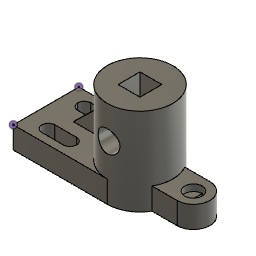
drawing_7 v1 (Autodesk Fusion 360 design; units mm, degrees)
Autodesk Fusion 360 part; units mm, degrees
sketch "Sketch10" plane through (0, 0, 0) normal (0, 1, 0) x (1, 0, 0)
  line L0 (15, -15) -> (101, -15)
  line L1 (101, -15) -> (101, -75)
  line L2 (101, -75) -> (15, -75)
  line L3 (15, -75) -> (15, -15)
  line L4 (15, -15) -> (150, -15)
  line L5 (135, -30) -> (90, -30)
  line L6 (90, -30) -> (90, -60)
  line L7 (90, -60) -> (135, -60)
  line L8 (150, -45) -> (150, -45)
  line L9 (135, -30) -> (150, -30)
  line L10 (135, -60) -> (150, -60)
  line L11 (165, -45) -> (165, -45)
  arc A0 (165, -45) -> (150, -30) centre (150, -45) ccw
  arc A1 (150, -60) -> (165, -45) centre (150, -45) ccw
  point P0 (150, -30)
  point P1 (150, -60)
  point P2 (165, -30)
  dimension "d50" = 86
  dimension "d51" = 60
  dimension "d59" = 135
  dimension "d60" = 60
  dimension "d61" = 30
  dimension "d64" = 30
  dimension "d65" = 15
  dimension "d66" = 15
  constraint horizontal L0
  constraint vertical L1
  constraint horizontal L2
  constraint vertical L3
  constraint perpendicular L3 L4
  constraint horizontal L5
  constraint vertical L6
  constraint horizontal L7
  constraint coincident P1 L7
  constraint coincident P0 L5
  constraint coincident P0 L8
  constraint horizontal L9
  constraint perpendicular L1 L10
  constraint coincident P2 L9
  constraint tangent L9 A0
  constraint tangent L10 A1
  measures "d50" distance of L0.start L0.end
  measures "d51" distance of L0.start L2.end
  measures "d59" distance of L0.start L4.end
  measures "d60" distance of P0 L5.end
  measures "d61" distance of P0 P1
  measures "d64" distance of L5.start P2
  measures "d65" radius of A0
  measures "d66" radius of A1
extrude "Extrude9" add sketch "Sketch10" along normal blind 20 contours L1 L5 L7 L9 L10 A0 A1 makes body 1
extrude "Extrude7" add sketch "Sketch10" along normal blind 20 separate body contours L0 L1 L2 L3 L4 L5 L6 L7 | L1 L5 L6 L7 makes body 2
sketch "Sketch11" plane through (0, 20, 0) normal (0, 1, 0) x (-1, 0, 0)
  line L0 (-15, 75) -> (-101, 75)
  line L1 (-101, 15) -> (-15, 15)
  line L2 (-15, 15) -> (-15, 75)
  circle A0 centre (-101, 45) radius 30
  line L3 (-101, 75) -> (-101, 15)
  dimension "d56" = 60
  measures "d56" diameter of A0
extrude "Extrude8" add sketch "Sketch11" along normal blind 60 contours A0 L3 | A0 L3 bodies 2
extrude "Extrude10" add 1 faces at (110.7493, 20, 47.2252) along direction (0, -1, 0) blind 20 on bodies 2 bodies 2 1
hole "Hole2" at (150, 20, 45) direction (0, -1, 0) diameter 16 depth 6 tip angle 180 bodies 2
sketch "Sketch12" plane through (0, 14, 0) normal (0, 1, 0) x (-1, 0, 0)
  circle A0 centre (-150, 45) radius 8
  line L0 (-150, 45) -> (-150, 37)
  line L1 (-150, 53) -> (-150, 44.4866)
  constraint coincident A0.centre L0.start
  constraint coincident A0 L0.end
  constraint vertical L0
  constraint coincident A0 L1.start
  constraint coincident L0 L1.end
  constraint parallel L0 L1
extrude "Extrude11" cut sketch "Sketch12" against normal blind 40 contours A0 L0 L1 picked at (-153.316, 49.1581) bodies 2
sketch "Sketch13" plane through (0, 80, 0) normal (0, 1, 0) x (-1, 0, 0)
  circle A0 centre (-101, 45) radius 30
  line L0 (-101, 45) -> (-91, 45)
  line L1 (-91, 45) -> (-91, 35)
  line L2 (-91, 35) -> (-101, 35)
  line L3 (-101, 35) -> (-101, 45)
  line L4 (-91, 35) -> (-111, 35)
  line L5 (-111, 35) -> (-111, 55)
  line L6 (-111, 55) -> (-91, 55)
  line L7 (-91, 55) -> (-91, 35)
  dimension "d76" = 10
  dimension "d77" = 10
  dimension "d78" = 20
  dimension "d79" = 20
  constraint horizontal L0
  constraint vertical L1
  constraint horizontal L2
  constraint vertical L3
  constraint coincident A0.centre L0.start
  constraint horizontal L4
  constraint vertical L5
  constraint horizontal L6
  constraint vertical L7
  measures "d76" distance of A0.centre L0.end
  measures "d77" distance of A0.centre L2.end
  measures "d78" distance of L1.end L4.end
  measures "d79" distance of L1.end L6.end
extrude "Extrude12" cut sketch "Sketch13" against normal blind 60 contours L0 L3 L4 L5 L6 L7 | L0 L1 L2 L3 L4 L7 bodies 2
sketch "Sketch14" plane through (0, 0, 55) normal (0, 0, -1) x (-1, 0, 0)
  line L0 (-91, 80) -> (-111, 80)
  line L1 (-111, 80) -> (-111, 20)
  line L2 (-111, 20) -> (-91, 20)
  line L3 (-91, 20) -> (-91, 80)
  line L4 (-101, 20) -> (-101, 80)
  circle A0 centre (-101, 50) radius 10
  dimension "d82" = 20
  constraint midpoint L2 L4.start
  constraint perpendicular L2 L4
  constraint midpoint L4 A0.centre
  measures "d82" diameter of A0
extrude "Extrude13" cut sketch "Sketch14" along normal blind 45 contours L4 A0 | L4 A0 bodies 2
hole "Hole3" at (101, 50, 55) direction (0, 0, 1) diameter 20 depth 30 tip angle 180 bodies 2
sketch "Sketch15" plane through (0, 20, 0) normal (0, 1, 0) x (-1, 0, 0)
  arc A0 (-101, 15) -> (-101, 75) centre (-101, 45) ccw
  line L0 (-101, 15) -> (-15, 15)
  line L1 (-15, 15) -> (-15, 75)
  line L2 (-15, 75) -> (-101, 75)
  line L3 (-15, 75) -> (-28, 75)
  line L4 (-34, 68) -> (-54, 68)
  line L5 (-60, 57) -> (-60, 57)
  line L6 (-54, 56) -> (-34, 56)
  line L7 (-28, 57) -> (-28, 57)
  arc A1 (-34, 56) -> (-28, 62) centre (-34, 62) ccw
  arc A2 (-28, 62) -> (-34, 68) centre (-34, 62) ccw
  arc A3 (-54, 68) -> (-60, 62) centre (-54, 62) ccw
  arc A4 (-60, 62) -> (-54, 56) centre (-54, 62) ccw
  line L8 (-32.9719, 22.0863) -> (-52.9796, 22.0863)
  line L9 (-58.9796, 28.0933) -> (-59, 28)
  line L10 (-53, 34) -> (-33, 34)
  line L11 (-27, 28) -> (-26.9719, 28.0754)
  arc A5 (-27, 28) -> (-33, 34) centre (-33, 28) ccw
  arc A6 (-32.9719, 22.0863) -> (-26.9719, 28.0754) centre (-32.9719, 28.0863) ccw
  arc A7 (-58.9796, 28.0933) -> (-52.9796, 22.0863) centre (-52.9796, 28.0863) ccw
  arc A8 (-53, 34) -> (-59, 28) centre (-53, 28) ccw
  point P0 (-28, 56)
  point P1 (-29.2024, 22.0863)
  point P2 (-27, 34)
  dimension "d92" = 6
  dimension "d93" = 6
  dimension "d94" = 6
  dimension "d95" = 6
  dimension "d100" = 6
  dimension "d101" = 6
  dimension "d102" = 6
  dimension "d103" = 6
  constraint coincident L1.end L2.start
  constraint perpendicular L1 L3
  constraint horizontal L4
  constraint horizontal L6
  constraint coincident P0 L6
  constraint tangent L6 A1
  constraint tangent L4 A2
  constraint tangent L4 A3
  constraint tangent L6 A4
  constraint horizontal L8
  constraint horizontal L10
  constraint coincident P2 L10
  constraint tangent L10 A5
  constraint coincident P1 L8
  constraint coincident P1 L11
  constraint tangent L8 A6
  constraint tangent L8 A7
  constraint tangent L10 A8
  measures "d92" radius of A1
  measures "d93" radius of A2
  measures "d94" radius of A3
  measures "d95" radius of A4
  measures "d100" radius of A5
  measures "d101" radius of A6
  measures "d102" radius of A7
  measures "d103" radius of A8
sketch "Sketch16" plane through (0, 20, 0) normal (0, 1, 0) x (-1, 0, 0)
  point P0 (-15, 75)
sketch "Sketch17" plane through (0, 20, 0) normal (0, 1, 0) x (-1, 0, 0)
  point P0 (-15, 15)
sketch "Sketch18" plane through (0, 20, 0) normal (0, 1, 0) x (-1, 0, 0)
extrude "Extrude14" cut sketch "Sketch15" against normal blind 55 contours L4 L6 A1 A2 A3 A4 | L8 L9 L10 L11 A5 A6 A7 A8 bodies 2
sketch "Sketch19" plane through (0, 20, 0) normal (0, 1, 0) x (-1, 0, 0)
  line L0 (-53, 34) -> (-33, 34)
  arc A0 (-27, 28) -> (-33, 34) centre (-33, 28) ccw
  line L1 (-27, 28) -> (-26.9719, 28.0754)
  arc A1 (-32.9719, 22.0863) -> (-26.9719, 28.0754) centre (-32.9719, 28.0863) ccw
  line L2 (-32.9719, 22.0863) -> (-52.9796, 22.0863)
  arc A2 (-58.9796, 28.0933) -> (-52.9796, 22.0863) centre (-52.9796, 28.0863) ccw
  line L3 (-58.9796, 28.0933) -> (-59, 28)
  arc A3 (-53, 34) -> (-59, 28) centre (-53, 28) ccw
  line L4 (-34, 56) -> (-54, 56)
  arc A4 (-54, 68) -> (-54, 56) centre (-54, 62) ccw
  line L5 (-54, 68) -> (-34, 68)
  arc A5 (-34, 56) -> (-34, 68) centre (-34, 62) ccw
  arc A6 (-101, 15) -> (-101, 75) centre (-101, 45) ccw
  line L6 (-101, 15) -> (-15, 15)
  line L7 (-15, 15) -> (-15, 75)
  line L8 (-15, 75) -> (-101, 75)
  line L9 (-15, 75) -> (-15, 45)
  line L10 (-15, 45) -> (-40, 45)
  line L11 (-40, 45) -> (-40, 39)
  line L12 (-40, 39) -> (-73.6757, 39)
  line L13 (-73.6757, 39) -> (-73.6757, 45)
  line L14 (-73.6757, 45) -> (-40, 45)
  line L15 (-40, 45) -> (-40, 39)
  dimension "d109" = 25
  dimension "d110" = 6
  constraint coincident L7.end L8.start
  constraint midpoint L7 L9.end
  constraint perpendicular L7 L10
  constraint perpendicular L10 L11
  constraint horizontal L12
  constraint vertical L13
  constraint horizontal L14
  constraint vertical L15
  measures "d109" distance of L9.end L10.end
  measures "d110" distance of L10.end L11.end
extrude "Extrude15" add sketch "Sketch19" along normal blind 30 contours A6 L11 L12 L14 L15 bodies 2
sketch "Sketch20" plane through (0, 0, 45) normal (0, 0, 1) x (1, 0, 0)
  line L0 (40, 20) -> (71, 20)
  line L1 (71, 20) -> (71, 50)
  line L2 (71, 50) -> (40, 50)
  line L3 (40, 50) -> (40, 20)
  line L4 (40, 20) -> (71, 50)
  constraint coincident L0.start L3.end
  constraint coincident L1.end L2.start
extrude "Extrude16" cut sketch "Sketch20" against normal blind 35 contours L2 L3 L4 bodies 2
